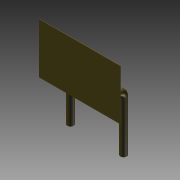
# Autodesk Inventor part: AS11CHtrh
Saved by Autodesk Inventor 2011 SP1 (Build 150282100, 282)
## iProperties
Created: 2018-06-01
Part Number: AS11CHtrh
Catalog Web Link: www.cadenas.de
Description: AS - Series - PC Terminals (H) - Poles 1 & 2-
Vendor: NKKSWITCHES
Document SubType Name: Modeling
Designer: psAdmin
Manufacturer: NKKSWITCHES
Mass: 0.00492183 g
Surface Area: 1.01703 cm^2
Volume: 0.00492183 cm^3
Density: 1 g/cm^3
Category: PARTsolutions
Company: NKKSWITCHES
Title: AS11CHtrh
Author: Cadenas PARTsolutions
PSOL_IDENT_0: {$CADENAS_DATA\23d-libs\nkkswitches\slides\as\parts\as_trmnls_h.prj},219 {VTYP=3D},{NB=AS11CHtrh},{L
PSOL_IDENT_1: INA=AS11CHtrh},{NN=AS - Series - PC Terminals (H) - Poles 1 & 2},{DATE=11.10.2017 10:53:50},{GEOMDAT
PSOL_IDENT_2: E=16.12.2008 13:46:00},{VERSION=},{LINEID=10},{LINESUBID=-1},{WBVAR=PLS,CRCTS,ACTU,TRMNLS}  {NB=AS11
PSOL_IDENT_3: CHtrh},{LINA=AS11CHtrh},{KT=DUMMY},{PN=AS11CH},{SRS=AS},{PLS=1},{CRCTS=1},{ACTU=C},{TRMNLS=H},{CRCTS
PSOL_IDENT_4: ALG=  '1', '1 - ON/NONE/OFF','2', '2 - ON/NONE/ON', '3', '3 - ON/OFF/ON' }
NN: AS - Series - PC Terminals (H) - Poles 1 & 2
NB: AS11CHtrh
NBSYN: $PN.trh
LINA: AS11CHtrh
PN: AS11CH
SRS: AS
PLS: 1 - SPST/SPDT
CRCTS: 1 - ON/NONE/OFF
ACTU: C - .150"(3,8mm)Long
TRMNLS: H - Right Angle with Bracket
SUPPLIER: NKKSWITCHES
ARTICLENO: AS11CHtrh
BOMINFO: AS11CHtrh
CREATOR: CADENAS GmbH
Autodesk Inventor part; units mm, degrees
sketch "Sketch_1" plane through (0, 0, 0) normal (0, 0, 1) x (1, 0, 0)
  line L0 (-3.8862, 2.413) -> (-3.8862, -2.413)
  line L1 (-3.8862, -2.413) -> (3.8862, -2.413)
  line L2 (3.8862, -2.413) -> (3.8862, 2.413)
  line L3 (3.8862, 2.413) -> (-3.8862, 2.413)
  constraints: 8 end point
extrude "Extrusion1" add sketch "Sketch_1" against normal blind 0.0254
sketch "Sketch_2" plane through (0, 0, -1.0414) normal (0, 0, 1) x (1, 0, 0)
  circle A0 centre (-2.54, -0.9906) radius 0.3048
  constraints: 1 centre point
extrude "Extrusion2" add sketch "Sketch_2" along normal blind 1.0414
sketch "Sketch_5" plane through (0, 0, -1.0414) normal (0, 0, 1) x (1, 0, 0)
  circle A0 centre (2.54, -0.9906) radius 0.3048
  constraints: 1 centre point
extrude "Extrusion3" add sketch "Sketch_5" along normal blind 1.0414
sketch "Sketch_6" plane through (0, 0, -1.0414) normal (0, 0, 1) x (1, 0, 0)
  line L0 (3.81, -1.6002) -> (-3.81, -1.6002)
  circle A0 centre (-2.54, -0.9906) radius 0.3048
  constraints: 2 end point, 1 centre point
revolve "Revolution1" add sketch "Sketch_6" angle 90 about axis through (3.81, -1.6002, -1.0414) along (-1, 0, 0)
sketch "Sketch_7" plane through (0, 0, -1.0414) normal (0, 0, 1) x (1, 0, 0)
  line L0 (2.54, -1.6002) -> (-2.54, -1.6002)
  circle A0 centre (2.54, -0.9906) radius 0.3048
  constraints: 2 end point, 1 centre point
revolve "Revolution2" add sketch "Sketch_7" angle 90 about axis through (2.54, -1.6002, -1.0414) along (-1, 0, 0)
sketch "Sketch_9" plane through (0, -1.6002, 0) normal (0, 1, 0) x (1, 0, 0)
  circle A0 centre (-2.54, 1.651) radius 0.3048
  constraints: 1 centre point
extrude "Extrusion4" add sketch "Sketch_9" against normal blind 4.826
sketch "Sketch_10" plane through (0, -1.6002, 0) normal (0, 1, 0) x (1, 0, 0)
  circle A0 centre (2.54, 1.651) radius 0.3048
  constraints: 1 centre point
extrude "Extrusion5" add sketch "Sketch_10" against normal blind 4.826
ref_plane "right_body_XY" through (0, 0, 0) normal (0, 0, -1) x (1, 0, 0)
ref_plane "right_body_YZ" through (0, 0, 0) normal (1, 0, 0) x (0, -1, 0)
ref_plane "right_body_ZX" through (0, 0, 0) normal (0, -1, 0) x (0, 0, -1)
body "Solid1"
